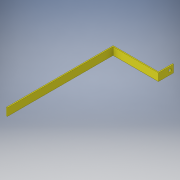
# Autodesk Inventor part: 1 x 6 x 16 x 1_8
Saved by Autodesk Inventor 2016 (Build 200138000, 138)
## iProperties
Created: 2015-06-18
Part Number: 1 x 6 x 16 x 1_8
Material: Aluminum 6061
Document SubType Name: Modeling
Designer: steele
Density: 2.7 g/cm^3
Appearance: Canary
Mass: 60.4981 g
Surface Area: 301.338 cm^2
Volume: 22.4067 cm^3
Author: steele
Autodesk Inventor part; units mm, degrees
ref_plane "YZ Plane" through (0, 0, 0) normal (1, 0, 0) x (0, 1, 0)
ref_plane "XZ Plane" through (0, 0, 0) normal (0, 1, 0) x (-1, 0, 0)
ref_plane "XY Plane" through (0, 0, 0) normal (0, 0, 1) x (1, 0, 0)
sketch "Sketch1" plane through (0, 0, 0) normal (0, 1, 0) x (-1, 0, 0)
  line L0 (0, 0) -> (0, 50.8)
  line L1 (0, 50.8) -> (152.4, 50.8)
  line L2 (152.4, 50.8) -> (152.4, 406.4)
  line L3 (152.4, 406.4) -> (155.575, 406.4)
  line L4 (155.575, 406.4) -> (155.575, 47.625)
  line L5 (155.575, 47.625) -> (3.175, 47.625)
  line L6 (3.175, 47.625) -> (3.175, 0)
  line L7 (3.175, 0) -> (0, 0)
  dimension "material_thickness" = 3.175
  dimension "d1" = 3.175
  dimension "d2" = 3.175
  dimension "total_length" = 406.4
  dimension "arm_length" = 152.4
  dimension "d5" = 50.8
  constraints: 16 end point, 7 perpendicular, 1 vertical
  measures "material_thickness" distance of L2.end L3.end
  measures "d1" distance between parallel lines of L5 L1
  measures "d2" distance of L6.end L0.start
  measures "total_length" vertical distance of L0.start L2.end
  measures "arm_length" distance from line of L0.end L2
  measures "d5" distance from line of L0.start L1
extrude "Extrusion1" add sketch "Sketch1" along normal mid plane 25.4
sketch "Sketch2" plane through (0, -12.7, 0) normal (1, 0, 0) x (0, 0, -1)
  line L0 (0, 12.7) -> (-50.8, 12.7) construction
  line L1 (-50.8, 25.4) -> (-50.8, 0) construction
  line L2 (-57.3367, 55.6538) -> (-54.5421, 53.2977) construction
  line L3 (-12.3225, 23.8478) -> (-12.3225, 1.5522) construction
  circle A0 centre (-12.3225, 12.7) radius 5.0165
  dimension "d8" = 10.033
  constraints: 6 end point, 2 midpoint, 1 centre point, 1 vertical
  measures "d8" diameter of A0
extrude "Extrusion2" cut sketch "Sketch2" against normal through all
equation "\"d1\" = material_thickness"
equation "\"d2\" = material_thickness"
body "Solid1"
